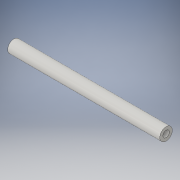
# Autodesk Inventor part: Delrin Spacer
Saved by Autodesk Inventor 2016 (Build 200138000, 138)
## iProperties
Created: 2018-05-10
Part Number: Delrin Spacer
Material: LCP Plastic
Document SubType Name: Modeling
Designer: Kade
Density: 1.626 g/cm^3
Appearance: White
Mass: 23.3208 g
Surface Area: 94.8127 cm^2
Volume: 14.3424 cm^3
Author: Kade
Autodesk Inventor part; units mm, degrees
ref_plane "YZ Plane" through (0, 0, 0) normal (1, 0, 0) x (0, 1, 0)
ref_plane "XZ Plane" through (0, 0, 0) normal (0, 1, 0) x (-1, 0, 0)
ref_plane "XY Plane" through (0, 0, 0) normal (0, 0, 1) x (1, 0, 0)
sketch "Sketch1" plane through (0, 0, 0) normal (1, 0, 0) x (0, 1, 0)
  circle A0 centre (0, 0) radius 3.2639
  circle A1 centre (0, 0) radius 6.35
  dimension "d0" = 6.5278
  dimension "d1" = 12.7
  constraints: 2 centre point, 2 coincident
  measures "d0" diameter of A0
  measures "d1" diameter of A1
extrude "Extrusion1" add sketch "Sketch1" along normal blind 153.8732
body "Solid1"
